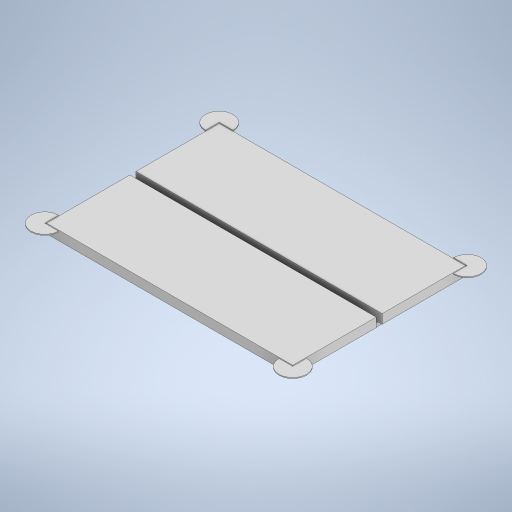
# Autodesk Inventor part: case_cover_v2
Saved by Autodesk Inventor 2023 (Build 270158000, 158)
## iProperties
Created: 2022-10-09
Part Number: case_cover_v2
Material: 일반
Document SubType Name: Modeling
Designer: 전상현
Density: 1 g/cm^3
Appearance: 기본값
Author: 전상현
Autodesk Inventor part; units mm, degrees
ref_plane "YZ Plane" through (0, 0, 0) normal (1, 0, 0) x (0, 1, 0)
ref_plane "XZ Plane" through (0, 0, 0) normal (0, 1, 0) x (-1, 0, 0)
sketch "스케치1" plane through (0, 0, 0) normal (0, 1, 0) x (-1, 0, 0)
  line L0 (64.8, -44.8) -> (-64.8, -44.8)
  line L1 (-64.8, -44.8) -> (-64.8, 44.8)
  line L2 (-64.8, 44.8) -> (64.8, 44.8)
  line L3 (64.8, 44.8) -> (64.8, -44.8)
  line L4 (64.8, -44.8) -> (-64.8, 44.8) construction
  line L5 (-64.8, -44.8) -> (64.8, 44.8) construction
  line L6 (64.8, -1.7) -> (-64.8, -1.7)
  line L7 (-64.8, -1.7) -> (-64.8, 1.7)
  line L8 (-64.8, 1.7) -> (64.8, 1.7)
  line L9 (64.8, 1.7) -> (64.8, -1.7)
  line L10 (64.8, -1.7) -> (-64.8, 1.7) construction
  line L11 (-64.8, -1.7) -> (64.8, 1.7) construction
  line L12 (27.5, 6.5) -> (-27.5, 6.5)
  line L13 (-27.5, 6.5) -> (-27.5, -3.5)
  line L14 (-27.5, -3.5) -> (27.5, -3.5)
  line L15 (27.5, -3.5) -> (27.5, 6.5)
  line L16 (-27.5, -3.5) -> (-24.5, -3.5)
  line L17 (-24.5, -3.5) -> (-24.5, 6.5)
  line L18 (-24.5, 6.5) -> (-27.5, 6.5)
  line L19 (-27.5, 6.5) -> (-27.5, -3.5)
  line L20 (27.5, -3.5) -> (24.5, -3.5)
  line L21 (24.5, -3.5) -> (24.5, 6.5)
  line L22 (24.5, 6.5) -> (27.5, 6.5)
  line L23 (27.5, 6.5) -> (27.5, -3.5)
  line L24 (25.5, -2.5) -> (20.1, -2.5)
  line L25 (20.1, -2.5) -> (20.1, 2.9)
  line L26 (20.1, 2.9) -> (25.5, 2.9)
  line L27 (25.5, 2.9) -> (25.5, -2.5)
  line L28 (13.6, -2.5) -> (13.6, 2.9)
  line L29 (19, -2.5) -> (13.6, -2.5)
  line L30 (19, 2.9) -> (19, -2.5)
  line L31 (13.6, 2.9) -> (19, 2.9)
  line L32 (7.1, -2.5) -> (7.1, 2.9)
  line L33 (12.5, -2.5) -> (7.1, -2.5)
  line L34 (12.5, 2.9) -> (12.5, -2.5)
  line L35 (7.1, 2.9) -> (12.5, 2.9)
  line L36 (0.6, -2.5) -> (0.6, 2.9)
  line L37 (6, -2.5) -> (0.6, -2.5)
  line L38 (6, 2.9) -> (6, -2.5)
  line L39 (0.6, 2.9) -> (6, 2.9)
  line L40 (-5.9, -2.5) -> (-5.9, 2.9)
  line L41 (-0.5, -2.5) -> (-5.9, -2.5)
  line L42 (-0.5, 2.9) -> (-0.5, -2.5)
  line L43 (-5.9, 2.9) -> (-0.5, 2.9)
  line L44 (-12.4, -2.5) -> (-12.4, 2.9)
  line L45 (-7, -2.5) -> (-12.4, -2.5)
  line L46 (-7, 2.9) -> (-7, -2.5)
  line L47 (-12.4, 2.9) -> (-7, 2.9)
  line L48 (-18.9, -2.5) -> (-18.9, 2.9)
  line L49 (-13.5, -2.5) -> (-18.9, -2.5)
  line L50 (-13.5, 2.9) -> (-13.5, -2.5)
  line L51 (-18.9, 2.9) -> (-13.5, 2.9)
  line L52 (-25.4, -2.5) -> (-25.4, 2.9)
  line L53 (-20, -2.5) -> (-25.4, -2.5)
  line L54 (-20, 2.9) -> (-20, -2.5)
  line L55 (-25.4, 2.9) -> (-20, 2.9)
  line L56 (27.5, 2.9) -> (-27.5, 2.9)
  line L57 (27.5, -2.5) -> (-27.5, -2.5)
  point P0 (0, 0)
  point P1 (0, 6.5)
  point P2 (-27.5, 2.9)
  point P3 (27.5, 2.9)
  dimension "d0" = 129.6
  dimension "d1" = 89.6
  dimension "d2" = 3.4
  dimension "d14" = 55
  dimension "d15" = 10
  dimension "d16" = 3
  dimension "d17" = 3
  dimension "d18" = 5.4
  dimension "d19" = 5.4
  dimension "d20" = 2
  dimension "d21" = 1
  dimension "d22" = 6.5
  dimension "d24" = 2.5
  constraints: 116 end point, 13 parallel, 9 point on line, 7 horizontal, 7 perpendicular, 5 midpoint, 1 vertical alignment, 56 other
  measures "d0" distance of L1.end L2.end
  measures "d1" distance of L0.end L1.end
  measures "d2" distance between parallel lines of L8 L6
  measures "d14" distance of L14.end L14.start
  measures "d15" distance of L12.end L14.start
  measures "d16" distance of L18.end L17.end
  measures "d17" distance of L21.end L22.end
  measures "d18" distance of L25.end L26.end
  measures "d19" distance of L25.start L25.end
  measures "d20" distance between parallel lines of L27 L15
  measures "d21" distance between parallel lines of L14 L24
  measures "d22" distance of L25.start L28.start
  measures "d24" distance from line of point (0, 0) L53
extrude "돌출3" add sketch "스케치1" along normal blind 2 contours L0 L1 L6 L13 L14 L15 L3 | L6 L15 L8 L3 | L1 L8 L13 L6 | L8 L15 L12 L13 L1 L2 L3 | L15 L14 L21 L24 L57 | L57 L53 L17 L14 L13 | L56 L26 L21 L12 L15 | L13 L12 L17 L55 L56 | L21 L14 L17 L53 L57 L49 L45 L41 L37 L33 L29 L24 | L26 L56 L31 L35 L39 L43 L47 L51 L55 L17 L12 L21
ref_plane "작업 평면1" through (0, 0, -2.5) normal (-1, 0, 0) x (0, 0, 1)
sketch "스케치6" plane through (0, 0, -2.5) normal (-1, 0, 0) x (0, 0, 1)
  line L0 (-1.2, 0) -> (-2.7, 0)
  line L1 (-2.7, 0) -> (-2.7, -4)
  line L2 (-2.7, -4) -> (-1.2, -4)
  line L3 (-1.2, -4) -> (-1.2, 0)
  line L4 (-2.7, -4) -> (2.3, -4)
  line L5 (2.3, -4) -> (2.3, -2.5)
  line L6 (2.3, -2.5) -> (-2.7, -2.5)
  line L7 (-2.7, -2.5) -> (-2.7, -4)
  point P0 (2.5, 0)
  point P1 (0, 0)
  point P2 (-1.2, -4)
  point P3 (-1.2, -2.5)
  dimension "d37" = 1.5
  dimension "d38" = 1.5
  dimension "d39" = 2.5
  dimension "d40" = 1.2
  dimension "d41" = 5
  constraints: 16 end point, 4 parallel, 2 horizontal, 2 perpendicular, 1 horizontal alignment
  measures "d37" distance of L2.end L1.end
  measures "d38" distance of L4.end L5.end
  measures "d39" distance between parallel lines of L0 L6
  measures "d40" distance of L0.start point (0, 0)
  measures "d41" distance between parallel lines of L1 L5
extrude "돌출5" add sketch "스케치6" along normal mid plane 20
fillet "모깎기1" radius 1.5 4 edges at (-10, 0, -4.45) (0, 0, -5.2) (10, 0, -4.45) (0, -4, -5.2)
sketch "스케치7" plane through (0, 2, 0) normal (0, 1, 0) x (1, 0, 0)
  line L0 (67, -47) -> (-67, -47)
  line L1 (-67, -47) -> (-67, 47)
  line L2 (-67, 47) -> (67, 47)
  line L3 (67, 47) -> (67, -47)
  line L4 (67, -47) -> (-67, 47) construction
  line L5 (-67, -47) -> (67, 47) construction
  line L6 (64.8, 44.8) -> (-64.8, 44.8) projected
  line L7 (-64.8, 44.8) -> (-64.8, -44.8) projected
  line L8 (-64.8, -44.8) -> (64.8, -44.8) projected
  line L9 (64.8, -44.8) -> (64.8, 44.8) projected
  line L10 (27.5, 2.5) -> (27.5, -2.9) projected
  line L11 (27.5, -2.9) -> (-27.5, -2.9) projected
  line L12 (-27.5, -2.9) -> (-27.5, 2.5) projected
  line L13 (-27.5, 2.5) -> (27.5, 2.5) projected
  line L14 (64.8, -44.8) -> (64.8, 44.8) projected
  line L15 (-67, -1.65) -> (67, -1.65)
  line L16 (67, -1.65) -> (67, 1.65)
  line L17 (67, 1.65) -> (-67, 1.65)
  line L18 (-67, 1.65) -> (-67, -1.65)
  line L19 (-67, -1.65) -> (67, 1.65) construction
  line L20 (67, -1.65) -> (-67, 1.65) construction
  point P0 (0, 0)
  point P1 (67, -2.9)
  point P2 (67, 2.5)
  point P3 (0, -2.9)
  point P4 (0, 2.5)
  dimension "d1" = 89.6
  dimension "d45" = 134
  dimension "d46" = 94
  dimension "d58" = 3.3
  constraints: 24 end point, 6 midpoint, 4 parallel, 3 point on line, 2 horizontal, 2 perpendicular
  measures "d45" distance of L1.end L2.end
  measures "d46" distance of L0.end L1.end
  measures "d58" distance between parallel lines of L17 L15
extrude "돌출6" add sketch "스케치7" along normal blind 5 contours L0 L1 L15 L7 L8 L9 L3 | L17 L9 L6 L7 L1 L2 L3 | L9 L8 L7 L15 L12 L11 L10 | L17 L10 L13 L12 L7 L6 L9 | L10 L11 L12 L15 | L17 L12 L13 L10
sketch "스케치8" plane through (0, 7, 0) normal (0, 1, 0) x (1, 0, 0)
  line L0 (67, 1.65) -> (67, 47) projected
  line L1 (67, 47) -> (-67, 47) projected
  line L2 (-67, 47) -> (-67, 1.65) projected
  line L3 (67.5, 47.5) -> (67.5, 2)
  line L4 (67.5, 2) -> (-67.5, 2)
  line L5 (-67.5, 2) -> (-67.5, 47.5)
  line L6 (-67.5, 47.5) -> (67.5, 47.5)
  circle A0 centre (67.5, 47.5) radius 7.5
  circle A1 centre (-67.5, 47.5) radius 7.5
  line L7 (-67, -47) -> (67, -47) projected
  line L8 (-67, 1.65) -> (67, 1.65) projected
  line L9 (67, -47) -> (67, -1.65) projected
  line L10 (67, -1.65) -> (-67, -1.65) projected
  line L11 (-67, -1.65) -> (-67, -47) projected
  point P0 (0, 0)
  point P1 (67.5, 40)
  point P2 (60, 47.5)
  point P3 (-60, 47.5)
  point P4 (-67.5, 40)
  dimension "d49" = 0.5
  dimension "d50" = 15
  dimension "d56" = 15
  constraints: 8 end point, 2 centre point, 2 coincident, 1 other
  measures "d49" distance between parallel lines of L0 L3
  measures "d50" diameter of A0
  measures "d56" diameter of A1
extrude "돌출7" add sketch "스케치8" against normal blind 0.5 contours L3 L6 A0 | A1 L6 L5
mirror "미러1" about plane through (0, 0, 0) normal (0, 0, 1) of "돌출7"
